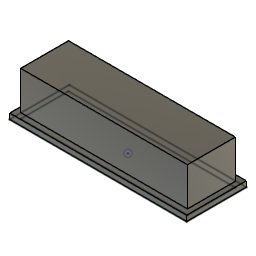
Door button support (Autodesk Fusion 360 archive; units mm, degrees)
design "Button"
Autodesk Fusion 360 part; units mm, degrees
sketch "Esquisse1" plane through (0, 0, 0) normal (0, 0, 1) x (1, 0, 0)
  line L0 (-30.5, 8.75) -> (30.5, 8.75)
  line L1 (30.5, 8.75) -> (30.5, -8.75)
  line L2 (30.5, -8.75) -> (-30.5, -8.75)
  line L3 (-30.5, -8.75) -> (-30.5, 8.75)
  line L4 (-32.35, 10.9) -> (32.35, 10.9)
  line L5 (32.35, 10.9) -> (32.35, -10.9)
  line L6 (32.35, -10.9) -> (-32.35, -10.9)
  line L7 (-32.35, -10.9) -> (-32.35, 10.9)
  dimension "d1" = 61
  dimension "d2" = 17.5
  dimension "d3" = 30.5
  dimension "d4" = 8.75
  dimension "d5" = 64.7
  dimension "d6" = 21.8
  dimension "d7" = 32.35
  dimension "d8" = 10.9
  constraint horizontal L0
  constraint vertical L1
  constraint horizontal L2
  constraint vertical L3
  constraint horizontal L4
  constraint vertical L5
  constraint horizontal L6
  constraint vertical L7
  measures "d1" distance of L0.start L0.end
  measures "d2" distance of L0.start L2.end
  measures "d3" horizontal distance of origin L0.start
  measures "d4" vertical distance of origin L0.start
  measures "d5" distance of L4.start L4.end
  measures "d6" distance of L4.start L6.end
  measures "d7" horizontal distance of origin L4.start
  measures "d8" vertical distance of origin L4.start
extrude "Extrusion1" add sketch "Esquisse1" along normal blind 16 contours L0 L1 L2 L3
extrude "Extrusion2" add sketch "Esquisse1" along normal blind 2
